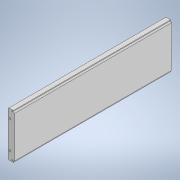
# Autodesk Inventor part: Case_Side
Saved by Autodesk Inventor 2022.2 (Build 262287010, 287A)
## iProperties
Created: 2024-11-06
Part Number: Case_Side
Material: Generisch
Document SubType Name: Modeling
Designer: ppovolni
Density: 1 g/cm^3
Appearance: Vorgabe
Author: ppovolni
Autodesk Inventor part; units mm, degrees
ref_plane "YZ Plane" through (0, 0, 0) normal (1, 0, 0) x (0, 1, 0)
ref_plane "XZ Plane" through (0, 0, 0) normal (0, 1, 0) x (-1, 0, 0)
ref_plane "XY Plane" through (0, 0, 0) normal (0, 0, 1) x (1, 0, 0)
sketch "Skizze1" plane through (0, 0, 0) normal (0, 0, 1) x (1, 0, 0)
  circle A0 centre (0, 0) radius 1.6
  circle A1 centre (0, 53) radius 1.6
  line L0 (-2.4, 69.5) -> (8.7, 69.5)
  line L1 (8.7, 69.5) -> (8.7, -16.5)
  line L2 (8.7, -16.5) -> (-2.4, -16.5)
  line L3 (-3.8, -15.1) -> (-3.8, 68.1)
  arc A2 (-2.4, 69.5) -> (-3.8, 68.1) centre (-2.4, 68.1) ccw
  arc A3 (-3.8, -15.1) -> (-2.4, -16.5) centre (-2.4, -15.1) ccw
  line L4 (3.5, 68) -> (8.7, 68)
  line L5 (8.7, 68) -> (8.7, 66.2)
  line L6 (8.7, 66.2) -> (3.5, 66.2)
  line L7 (3.5, 66.2) -> (3.5, 68)
  line L8 (6.2, 69.5) -> (8.7, 69.5)
  line L9 (8.7, 69.5) -> (8.7, 68)
  line L10 (8.7, 68) -> (6.2, 68)
  line L11 (6.2, 68) -> (6.2, 69.5)
  line L12 (8.7, -12.7) -> (3.5, -12.7)
  line L13 (3.5, -12.7) -> (3.5, -14.5)
  line L14 (3.5, -14.5) -> (8.7, -14.5)
  line L15 (8.7, -14.5) -> (8.7, -12.7)
  line L16 (6.2, -14.5) -> (8.7, -14.5)
  line L17 (8.7, -14.5) -> (8.7, -16.5)
  line L18 (8.7, -16.5) -> (6.2, -16.5)
  line L19 (6.2, -16.5) -> (6.2, -14.5)
  point P0 (-3.8, 69.5)
  point P1 (-3.8, -16.5)
  point P2 (6.2, 68.75)
  point P3 (7.45, -16.5)
  point P4 (7.45, -14.5)
  dimension "d0" = 3.2
  dimension "d1" = 12.5
  dimension "d2" = 86
  dimension "d3" = 16.5
  dimension "d4" = 16.5
  dimension "d5" = 3.8
  dimension "d6" = 1.4
  dimension "d7" = 2.5
  dimension "d8" = 5.2
  dimension "d9" = 1.5
  dimension "d10" = 1.8
  dimension "d11" = 5.2
  dimension "d12" = 1.8
  dimension "d14" = 2.5
  dimension "d15" = 2
  constraints: 40 end point, 10 parallel, 8 point on line, 5 horizontal, 5 perpendicular, 4 centre point, 4 point on circle, 4 tangent, 3 midpoint, 2 collinear, 2 equal radius, 1 coincident, 1 vertical alignment
  measures "d0" diameter of A1
  measures "d1" distance of point (-3.8, 69.5) L0.end
  measures "d2" distance of point (-3.8, -16.5) point (-3.8, 69.5)
  measures "d3" distance from line of A1.centre L0
  measures "d4" distance from line of L2 point (0, 0)
  measures "d5" distance from line of L3 A1.centre
  measures "d6" radius of A2
  measures "d7" distance from line of L9 point (6.2, 68.75)
  measures "d8" distance between parallel lines of L1 L7
  measures "d9" distance between parallel lines of L10 L0
  measures "d10" distance of L6.end L4.start
  measures "d11" distance of L12.start L12.end
  measures "d12" distance of L12.end L13.end
  measures "d14" distance between parallel lines of L19 L1
  measures "d15" distance of point (7.45, -16.5) point (7.45, -14.5)
extrude "Extrusion1" add sketch "Skizze1" along normal blind 300 contours L0 L11 L4 L7 L6 L1 L12 L13 L14 L19 L2 A3 L3 A2
